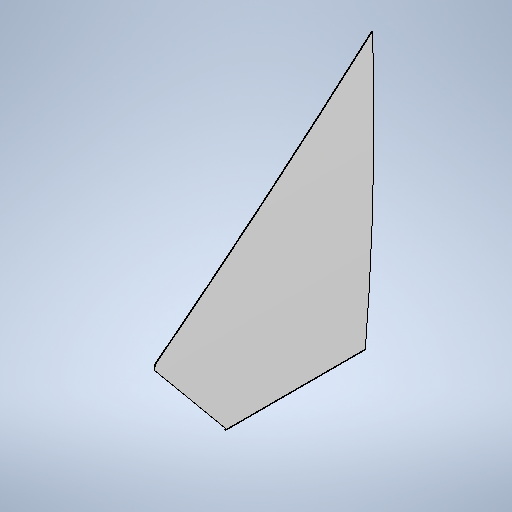
# Autodesk Inventor part: MSC 311 SHEET LEFT BOARD FACE
Saved by Autodesk Inventor 2025 (Build 290162010, 162A)
## iProperties
Created: 2024-04-18
Part Number: MSC 311 SHEET LEFT BOARD FACE
Material: AISI304
Document SubType Name: Sheet Metal
Designer: admin
Stock Number: МОО 311 лист левый борт морда
Mass: 19260 g
Surface Area: 16165.6 cm^2
Volume: 2407.5 cm^3
Density: 8 g/cm^3
Sheet Metal Rule: AISI304 3mm Die 32
Sheet Metal Width: 980,000 mm
Sheet Metal Length: 1329,475 mm
Sheet Metal Area: 1302885,200 mm^2
Appearance: Default
Flat Pattern Width: 98 cm
Flat Pattern Length: 132.947 cm
Flat Pattern Area: 13028.9 cm^2
Author: admin
Autodesk Inventor part; units mm, degrees
ref_plane "YZ Plane" through (0, 0, 0) normal (1, 0, 0) x (0, 1, 0)
ref_plane "XZ Plane" through (0, 0, 0) normal (0, 1, 0) x (-1, 0, 0)
ref_plane "XY Plane" through (0, 0, 0) normal (0, 0, 1) x (1, 0, 0)
sketch "Sketch1" plane through (0, 0, 0) normal (0, 0, 1) x (1, 0, 0)
  line L0 (394.757121, -1035.809004) -> (394.757121, -1085.809004) construction
  line L1 (0, -1088.809004) -> (0, -1878.848599) construction
  arc A0 (0.156692, -1876.974279) -> (0, -35.848599) centre (-11011.509331, -957.348599) ccw
  arc A1 (0, -1878.848599) -> (0.156692, -1876.974279) centre (-11011.509331, -957.348599) ccw construction
  arc A2 (-1.35267, -1880.154857) -> (0.156692, -1876.974279) centre (-4.825962, -1876.558158) ccw
  line L2 (-1.35267, -1880.154857) -> (0, -1878.848599) construction
  line L3 (-45.318407, -1922.612076) -> (-1.35267, -1880.154857)
  line L4 (0, -1878.848599) -> (0, 0) construction
  line L5 (0, -1878.848599) -> (1.880433, -1878.848599) construction
  line L6 (0, -35.848599) -> (0, -35.848599) construction
  dimension "d153" = 5
  dimension "d154" = 63
  dimension "d155" = 11050
  dimension "d156" = 136
  dimension "d174" = 1843
  dimension "d175" = 0
  measures "d153" radius of A2
  measures "d154" distance of L1.end L3.start
  measures "d155" radius of A0
  measures "d156" angle of L2 L5
  measures "d174" distance from line of point (0, -1878.849) L6
  measures "d175" distance of L6.start L6.end
contour flange "Contour Flange2" sketch "Sketch1" thickness 3 bend radius 5 width 980 along (0, 0, 1) mid plane no both sides no wall seen from (-23.335539, -1901.383467, 0) lies toward (0.6946584, -0.7193398, 0) curves L3 A2 A0
bend "Bend2"
corner "Corner2"
sketch "Sketch2" plane through (0, 0, 0) normal (1, 0, 0) x (0, 1, 0)
  line L0 (-1877.223951, 980) -> (-1877.223951, 0) construction
  line L1 (-1877.223951, 0) -> (-35.598418, 0)
  line L2 (-35.598418, 0) -> (-35.598418, 980)
  line L3 (-1877.223951, 980) -> (-35.598418, 980)
  line L4 (-1882.312877, 980) -> (-1882.312877, 0) construction
  line L5 (-1924.770096, 980) -> (-1882.312877, 980)
  line L6 (-1924.770096, 0) -> (-1924.770096, 980)
  line L7 (-1924.770096, 0) -> (-1882.312877, 0)
  line L8 (-1877.223951, 980) -> (-1882.312877, 980)
  line L9 (-1877.223951, 0) -> (-1882.312877, 0)
  line L10 (-613.598418, 0) -> (-1435.916056, 980)
  line L11 (-1458.052948, 980) -> (-1924.770096, 588.377813)
  line L12 (-614.437518, 0) -> (-614.437518, 1)
  point P0 (0, 0)
  dimension "d160" = 300
  dimension "d162" = 40
  dimension "d163" = 40
  dimension "d172" = 578
  dimension "d176" = 1
  constraints: 10 end point, 6 point on line, 1 collinear, 1 perpendicular, 1 vertical
  measures "d160" distance from line of L11 L5.start
  measures "d162" angle of L3 L11
  measures "d163" angle of L2 L10
  measures "d172" distance of L10.start L1.end
  measures "d176" distance of L12.start L12.end
extrude "Extrusion2" cut sketch "Sketch2" along normal through all both and the other way through all contours L12 L10 L1 | L10 L3 L2 L1 | L6 L5 L8 L3 L11
sketch "Sketch6" plane through (-1.35267, -1880.154857, 625.814443) normal (-0.6946584, 0.7193398, 0) x (0.7193398, 0.6946584, 0)
  line L0 (-43.900854, 36.326501) -> (-43.900854, 205.720848) construction
  line L1 (-43.900854, 205.720848) -> (-29.383925, 205.720848) construction
  line L2 (-29.383925, 205.720848) -> (-29.383925, 36.326501) construction
  line L3 (-29.383925, 36.326501) -> (-43.900854, 36.326501) construction
  point P0 (1307.038339, 625.814443)
  constraints: 2 other
mark "Mark4"
equation "\"d36\" = Thickness"
equation "\"d37\" = BendReliefWidth"
equation "\"d38\" = BendReliefDepth"
equation "\"d39\" = MinimumRemnant"
equation "\"d40\" = TransitionRadius"
equation "\"d42\" = BendRadius"
equation "\"d44\" = CornerReliefSize"
equation "\"d45\" = GapSize"
equation "\"d46\" = JacobiRadiusSize"
equation "\"BendReliefWidth\" = Thickness"
equation "\"BendReliefDepth\" = 0.5 * Thickness"
equation "\"CornerReliefSize\" = 4 * Thickness"
equation "\"MinimumRemnant\" = 2 * Thickness"
equation "\"GapSize\" = Thickness"
equation "\"Thickness\" = 3"
equation "\"TransitionRadius\" = 5"
equation "\"BendRadius\" = 5"
equation "\"JacobiRadiusSize\" = 5"
body "Solid3"
